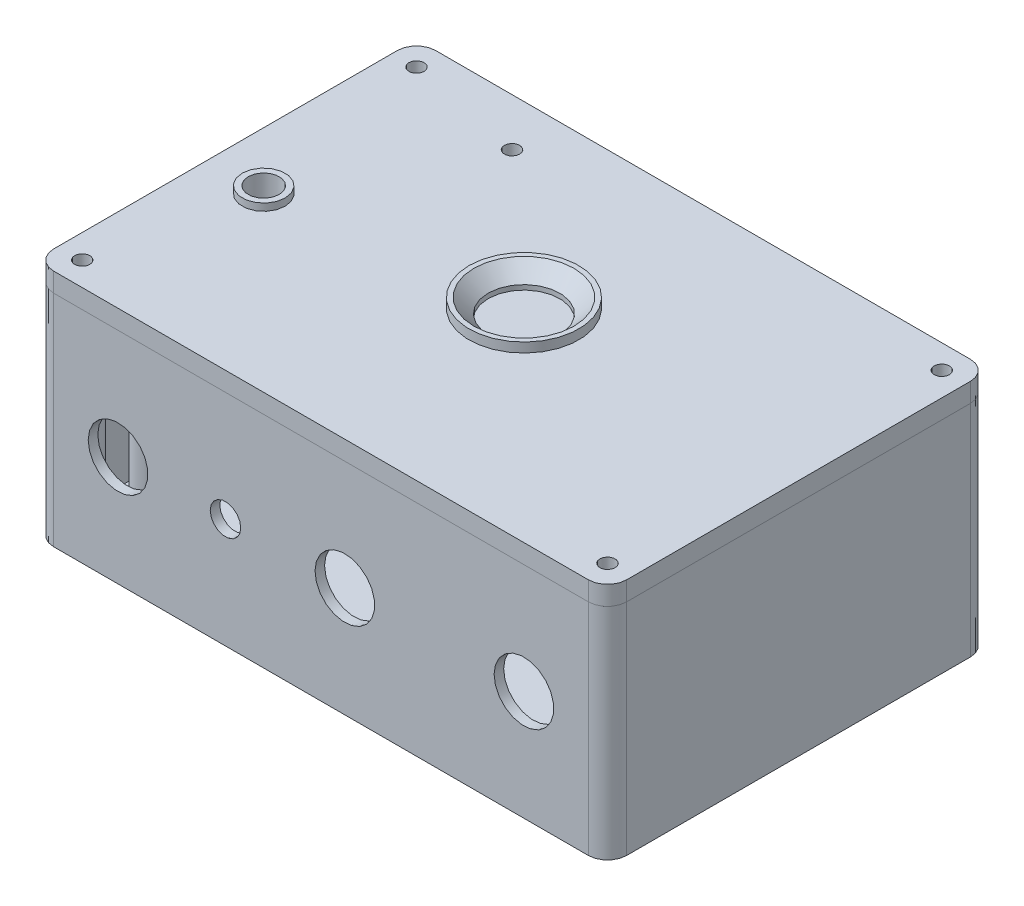
GridUp-Kutu (Autodesk Fusion 360 design; units mm, degrees)
part number: 2026-09-14-07-36-03-763
Autodesk Fusion 360 part; units mm, degrees
sketch "Çizim1" plane through (0, 0, 0) normal (0, 0, 1) x (1, 0, 0)
  line L0 (0, 0) -> (120, 0)
  line L1 (120, 0) -> (120, 80)
  line L2 (120, 80) -> (0, 80)
  line L3 (0, 80) -> (0, 0)
sketch "Çizim2" plane through (0, 0, 0) normal (0, 0, 1) x (1, 0, 0)
  circle A0 centre (5, 5) radius 3.5
  circle A1 centre (115, 5) radius 3.5
  circle A2 centre (5, 75) radius 3.5
  circle A3 centre (115, 75) radius 3.5
ref_plane "WorkPlane1" through (0, 0, 46) normal (0, 0, 1) x (1, 0, 0)
sketch "Çizim3" plane through (0, 0, 46) normal (0, 0, 1) x (1, 0, 0)
  line L0 (0, 0) -> (120, 0)
  line L1 (120, 0) -> (120, 80)
  line L2 (120, 80) -> (0, 80)
  line L3 (0, 80) -> (0, 0)
ref_plane "WorkPlane2" through (0, 0, 50) normal (0, 0, 1) x (1, 0, 0)
sketch "Çizim4" plane through (0, 0, 50) normal (0, 0, 1) x (1, 0, 0)
  circle A0 centre (60, 42.5) radius 11.5
sketch "Çizim5" plane through (0, 0, 50) normal (0, 0, 1) x (1, 0, 0)
  circle A0 centre (60, 42.5) radius 7.5
sketch "Çizim6" plane through (0, 0, 50) normal (0, 0, 1) x (1, 0, 0)
  circle A0 centre (12, 36) radius 4.5
sketch "Çizim7" plane through (0, 0, 50) normal (0, 0, 1) x (1, 0, 0)
  circle A0 centre (12, 36) radius 3.25
extrude "Ekstrüzyon7" cut sketch "Çizim7" along normal mid plane 16
sketch "Çizim8" plane through (0, 0, 50) normal (0, 0, 1) x (1, 0, 0)
  circle A0 centre (30, 70) radius 1.6
extrude "Ekstrüzyon8" cut sketch "Çizim8" along normal mid plane 16
sketch "Çizim9" plane through (0, 0, 50) normal (0, 0, 1) x (1, 0, 0)
  circle A0 centre (5, 5) radius 1.6
  circle A1 centre (115, 5) radius 1.6
  circle A2 centre (5, 75) radius 1.6
  circle A3 centre (115, 75) radius 1.6
extrude "Ekstrüzyon9" cut sketch "Çizim9" along normal mid plane 16
sketch "Çizim10" plane through (0, 0, 50) normal (0, 0, 1) x (1, 0, 0)
  circle A0 centre (5, 5) radius 1.25
  circle A1 centre (115, 5) radius 1.25
  circle A2 centre (5, 75) radius 1.25
  circle A3 centre (115, 75) radius 1.25
ref_plane "WorkPlane3" through (0, 0, 47.5) normal (0, 0, 1) x (1, 0, 0)
sketch "Çizim11" plane through (0, 0, 47.5) normal (0, 0, 1) x (1, 0, 0)
  circle A0 centre (60, 42.5) radius 7.5
sketch "Çizim12" plane through (0, 0, 0) normal (0, 1, 0) x (1, 0, 0)
  circle A0 centre (17.5, -23) radius 6.25
  circle A1 centre (47.5, -23) radius 5.5
  circle A2 centre (75, -23) radius 5.5
  circle A3 centre (102.5, -23) radius 3.2
sketch "Çizim13" plane through (0, 0, 0) normal (0, 0, 1) x (1, 0, 0)
  line L0 (12.75, 42.5) -> (22.25, 42.5)
  arc A0 (22.25, 42.5) -> (22.25, 48) centre (22.25, 45.25) ccw
  line L1 (22.25, 48) -> (12.75, 48)
  arc A1 (12.75, 48) -> (12.75, 42.5) centre (12.75, 45.25) ccw
  line L2 (97.75, 42.5) -> (107.25, 42.5)
  arc A2 (107.25, 42.5) -> (107.25, 48) centre (107.25, 45.25) ccw
  line L3 (107.25, 48) -> (97.75, 48)
  arc A3 (97.75, 48) -> (97.75, 42.5) centre (97.75, 45.25) ccw
sketch "Çizim14" plane through (0, 0, 0) normal (0, 0, 1) x (1, 0, 0)
  circle A0 centre (7.5, 7.5) radius 3.5
  circle A1 centre (112.5, 7.5) radius 3.5
  circle A2 centre (7.5, 72.5) radius 3.5
  circle A3 centre (112.5, 72.5) radius 3.5
sketch "Çizim15" plane through (0, 0, 0) normal (0, 0, 1) x (1, 0, 0)
  line L0 (42.5, 20) -> (77.5, 20)
  line L1 (77.5, 20) -> (77.5, 62)
  line L2 (77.5, 62) -> (42.5, 62)
  line L3 (42.5, 62) -> (42.5, 20)
ref_plane "WorkPlane4" through (0, 0, -5) normal (0, 0, 1) x (1, 0, 0)
sketch "Çizim16" plane through (0, 0, -5) normal (0, 0, 1) x (1, 0, 0)
  line L0 (42.5, 23.25) -> (77.5, 23.25)
  line L1 (77.5, 23.25) -> (77.5, 58.75)
  line L2 (77.5, 58.75) -> (42.5, 58.75)
  line L3 (42.5, 58.75) -> (42.5, 23.25)
sketch "Çizim17" plane through (0, 0, 0) normal (0, 0, 1) x (1, 0, 0)
  line L0 (0, 0) -> (120, 0)
  line L1 (120, 0) -> (120, 80)
  line L2 (120, 80) -> (0, 80)
  line L3 (0, 80) -> (0, 0)
sketch "Çizim18" plane through (0, 0, 0) normal (0, 0, 1) x (1, 0, 0)
  circle A0 centre (5, 5) radius 3.5
  circle A1 centre (115, 5) radius 3.5
  circle A2 centre (5, 75) radius 3.5
  circle A3 centre (115, 75) radius 3.5
sketch "Çizim19" plane through (0, 0, 0) normal (0, 0, 1) x (1, 0, 0)
  circle A0 centre (12, 12) radius 3
  circle A1 centre (108, 12) radius 3
  circle A2 centre (12, 68) radius 3
  circle A3 centre (108, 68) radius 3
ref_plane "WorkPlane5" through (0, 0, 39.4) normal (0, 0, 1) x (1, 0, 0)
sketch "Çizim20" plane through (0, 0, 39.4) normal (0, 0, 1) x (1, 0, 0)
  circle A0 centre (12, 12) radius 1.25
  circle A1 centre (108, 12) radius 1.25
  circle A2 centre (12, 68) radius 1.25
  circle A3 centre (108, 68) radius 1.25
ref_plane "WorkPlane6" through (0, 0, 46) normal (0, 0, 1) x (1, 0, 0)
sketch "Çizim21" plane through (0, 0, 46) normal (0, 0, 1) x (1, 0, 0)
  line L0 (0, 0) -> (120, 0)
  line L1 (120, 0) -> (120, 80)
  line L2 (120, 80) -> (0, 80)
  line L3 (0, 80) -> (0, 0)
extrude "Ekstrüzyon21" add sketch "Çizim21" along normal blind 4 separate body makes body 1
fillet "Radyus4" radius 4 4 edges at (0, 80, 48) (120, 80, 48) (120, 0, 48) (0, 0, 48) on bodies 1
ref_plane "WorkPlane7" through (0, 0, 50) normal (0, 0, 1) x (1, 0, 0)
sketch "Çizim22" plane through (0, 0, 50) normal (0, 0, 1) x (1, 0, 0)
  circle A0 centre (60, 42.5) radius 11.5
extrude "Ekstrüzyon22" add sketch "Çizim22" along normal blind 2 bodies 1
sketch "Çizim23" plane through (0, 0, 50) normal (0, 0, 1) x (1, 0, 0)
  circle A0 centre (60, 42.5) radius 7.5
extrude "Ekstrüzyon23" cut sketch "Çizim23" along normal mid plane 16 bodies 1
chamfer "Pah2" distance 3 angle 45 1 edges at (53.0075, 45.2121, 52) tangent chain off on bodies 1
sketch "Çizim24" plane through (0, 0, 50) normal (0, 0, 1) x (1, 0, 0)
  circle A0 centre (12, 36) radius 4.5
extrude "Ekstrüzyon24" add sketch "Çizim24" along normal blind 1.5 bodies 1
sketch "Çizim25" plane through (0, 0, 50) normal (0, 0, 1) x (1, 0, 0)
  circle A0 centre (12, 36) radius 3.25
extrude "Ekstrüzyon25" cut sketch "Çizim25" along normal mid plane 16 bodies 1
sketch "Çizim26" plane through (0, 0, 50) normal (0, 0, 1) x (1, 0, 0)
  circle A0 centre (30, 70) radius 1.6
extrude "Ekstrüzyon26" cut sketch "Çizim26" along normal mid plane 16 bodies 1
sketch "Çizim27" plane through (0, 0, 50) normal (0, 0, 1) x (1, 0, 0)
  circle A0 centre (5, 5) radius 1.6
  circle A1 centre (115, 5) radius 1.6
  circle A2 centre (5, 75) radius 1.6
  circle A3 centre (115, 75) radius 1.6
extrude "Ekstrüzyon27" cut sketch "Çizim27" along normal mid plane 16 bodies 1
sketch "Çizim28" plane through (0, 0, 50) normal (0, 0, 1) x (1, 0, 0)
  circle A0 centre (5, 5) radius 1.25
  circle A1 centre (115, 5) radius 1.25
  circle A2 centre (5, 75) radius 1.25
  circle A3 centre (115, 75) radius 1.25
ref_plane "WorkPlane8" through (0, 0, 47.5) normal (0, 0, 1) x (1, 0, 0)
sketch "Çizim29" plane through (0, 0, 47.5) normal (0, 0, 1) x (1, 0, 0)
  circle A0 centre (60, 42.5) radius 7.5
sketch "Çizim30" plane through (0, 0, 0) normal (0, 1, 0) x (1, 0, 0)
  circle A0 centre (17.5, -23) radius 6.25
  circle A1 centre (47.5, -23) radius 5.5
  circle A2 centre (75, -23) radius 5.5
  circle A3 centre (102.5, -23) radius 3.2
sketch "Çizim31" plane through (0, 0, 0) normal (0, 0, 1) x (1, 0, 0)
  line L0 (12.75, 42.5) -> (22.25, 42.5)
  arc A0 (22.25, 42.5) -> (22.25, 48) centre (22.25, 45.25) ccw
  line L1 (22.25, 48) -> (12.75, 48)
  arc A1 (12.75, 48) -> (12.75, 42.5) centre (12.75, 45.25) ccw
  line L2 (97.75, 42.5) -> (107.25, 42.5)
  arc A2 (107.25, 42.5) -> (107.25, 48) centre (107.25, 45.25) ccw
  line L3 (107.25, 48) -> (97.75, 48)
  arc A3 (97.75, 48) -> (97.75, 42.5) centre (97.75, 45.25) ccw
sketch "Çizim32" plane through (0, 0, 0) normal (0, 0, 1) x (1, 0, 0)
  circle A0 centre (7.5, 7.5) radius 3.5
  circle A1 centre (112.5, 7.5) radius 3.5
  circle A2 centre (7.5, 72.5) radius 3.5
  circle A3 centre (112.5, 72.5) radius 3.5
sketch "Çizim33" plane through (0, 0, 0) normal (0, 0, 1) x (1, 0, 0)
  line L0 (42.5, 20) -> (77.5, 20)
  line L1 (77.5, 20) -> (77.5, 62)
  line L2 (77.5, 62) -> (42.5, 62)
  line L3 (42.5, 62) -> (42.5, 20)
ref_plane "WorkPlane9" through (0, 0, -5) normal (0, 0, 1) x (1, 0, 0)
sketch "Çizim34" plane through (0, 0, -5) normal (0, 0, 1) x (1, 0, 0)
  line L0 (42.5, 23.25) -> (77.5, 23.25)
  line L1 (77.5, 23.25) -> (77.5, 58.75)
  line L2 (77.5, 58.75) -> (42.5, 58.75)
  line L3 (42.5, 58.75) -> (42.5, 23.25)
sketch "Çizim35" plane through (0, 0, 0) normal (0, 0, 1) x (1, 0, 0)
  line L0 (0, 0) -> (120, 0)
  line L1 (120, 0) -> (120, 80)
  line L2 (120, 80) -> (0, 80)
  line L3 (0, 80) -> (0, 0)
extrude "Ekstrüzyon35" add sketch "Çizim35" along normal blind 46 separate body makes body 2
fillet "Radyus5" radius 4 4 edges at (0, 80, 23) (120, 80, 23) (120, 0, 23) (0, 0, 23) on bodies 2
shell "Kabuk3" thickness 2 removed faces 1 at (78.6667, 26.6667, 46) on bodies 2
sketch "Çizim36" plane through (0, 0, 0) normal (0, 0, 1) x (1, 0, 0)
  circle A0 centre (5, 5) radius 3.5
  circle A1 centre (115, 5) radius 3.5
  circle A2 centre (5, 75) radius 3.5
  circle A3 centre (115, 75) radius 3.5
extrude "Ekstrüzyon36" add sketch "Çizim36" along normal blind 46 bodies 2
sketch "Çizim37" plane through (0, 0, 0) normal (0, 0, 1) x (1, 0, 0)
  circle A0 centre (12, 12) radius 3
  circle A1 centre (108, 12) radius 3
  circle A2 centre (12, 68) radius 3
  circle A3 centre (108, 68) radius 3
extrude "Ekstrüzyon37" add sketch "Çizim37" along normal blind 39.4 bodies 2
ref_plane "WorkPlane10" through (0, 0, 39.4) normal (0, 0, 1) x (1, 0, 0)
sketch "Çizim38" plane through (0, 0, 39.4) normal (0, 0, 1) x (1, 0, 0)
  circle A0 centre (12, 12) radius 1.25
  circle A1 centre (108, 12) radius 1.25
  circle A2 centre (12, 68) radius 1.25
  circle A3 centre (108, 68) radius 1.25
extrude "Ekstrüzyon38" cut sketch "Çizim38" against normal blind 8 bodies 2
ref_plane "WorkPlane11" through (0, 0, 46) normal (0, 0, 1) x (1, 0, 0)
sketch "Çizim39" plane through (0, 0, 46) normal (0, 0, 1) x (1, 0, 0)
  line L0 (0, 0) -> (120, 0)
  line L1 (120, 0) -> (120, 80)
  line L2 (120, 80) -> (0, 80)
  line L3 (0, 80) -> (0, 0)
extrude "Ekstrüzyon39" add sketch "Çizim39" along normal blind 4 separate body makes body 3
fillet "Radyus6" radius 4 4 edges at (0, 80, 48) (120, 80, 48) (120, 0, 48) (0, 0, 48) on bodies 3
ref_plane "WorkPlane12" through (0, 0, 50) normal (0, 0, 1) x (1, 0, 0)
sketch "Çizim40" plane through (0, 0, 50) normal (0, 0, 1) x (1, 0, 0)
  circle A0 centre (60, 42.5) radius 11.5
extrude "Ekstrüzyon40" add sketch "Çizim40" along normal blind 2 bodies 3
sketch "Çizim41" plane through (0, 0, 50) normal (0, 0, 1) x (1, 0, 0)
  circle A0 centre (60, 42.5) radius 7.5
extrude "Ekstrüzyon41" cut sketch "Çizim41" along normal mid plane 16 bodies 3
chamfer "Pah3" distance 3 angle 45 1 edges at (53.0075, 45.2121, 52) tangent chain off on bodies 3
sketch "Çizim42" plane through (0, 0, 50) normal (0, 0, 1) x (1, 0, 0)
  circle A0 centre (12, 36) radius 4.5
extrude "Ekstrüzyon42" add sketch "Çizim42" along normal blind 1.5 bodies 3
sketch "Çizim43" plane through (0, 0, 50) normal (0, 0, 1) x (1, 0, 0)
  circle A0 centre (12, 36) radius 3.25
extrude "Ekstrüzyon43" cut sketch "Çizim43" along normal mid plane 16 bodies 3
sketch "Çizim44" plane through (0, 0, 50) normal (0, 0, 1) x (1, 0, 0)
  circle A0 centre (30, 70) radius 1.6
extrude "Ekstrüzyon44" cut sketch "Çizim44" along normal mid plane 16 bodies 3
sketch "Çizim45" plane through (0, 0, 50) normal (0, 0, 1) x (1, 0, 0)
  circle A0 centre (5, 5) radius 1.6
  circle A1 centre (115, 5) radius 1.6
  circle A2 centre (5, 75) radius 1.6
  circle A3 centre (115, 75) radius 1.6
extrude "Ekstrüzyon45" cut sketch "Çizim45" along normal mid plane 16 bodies 3
sketch "Çizim46" plane through (0, 0, 50) normal (0, 0, 1) x (1, 0, 0)
  circle A0 centre (5, 5) radius 1.25
  circle A1 centre (115, 5) radius 1.25
  circle A2 centre (5, 75) radius 1.25
  circle A3 centre (115, 75) radius 1.25
extrude "Ekstrüzyon46" cut sketch "Çizim46" against normal blind 16 bodies 2
ref_plane "WorkPlane13" through (0, 0, 47.5) normal (0, 0, 1) x (1, 0, 0)
sketch "Çizim47" plane through (0, 0, 47.5) normal (0, 0, 1) x (1, 0, 0)
  circle A0 centre (60, 42.5) radius 7.5
extrude "Ekstrüzyon47" add sketch "Çizim47" along normal mid plane 1 separate body makes body 4
sketch "Çizim48" plane through (0, 0, 0) normal (0, 1, 0) x (1, 0, 0)
  circle A0 centre (17.5, -23) radius 6.25
  circle A1 centre (40, -23) radius 3.2
  circle A2 centre (65, -23) radius 6.25
  circle A3 centre (102.5, -23) radius 6.25
extrude "Ekstrüzyon48" cut sketch "Çizim48" along normal mid plane 6 bodies 2
sketch "Çizim49" plane through (0, 0, 0) normal (0, 0, 1) x (1, 0, 0)
  line L0 (12.75, 42.5) -> (22.25, 42.5)
  arc A0 (22.25, 42.5) -> (22.25, 48) centre (22.25, 45.25) ccw
  line L1 (22.25, 48) -> (12.75, 48)
  arc A1 (12.75, 48) -> (12.75, 42.5) centre (12.75, 45.25) ccw
  line L2 (97.75, 42.5) -> (107.25, 42.5)
  arc A2 (107.25, 42.5) -> (107.25, 48) centre (107.25, 45.25) ccw
  line L3 (107.25, 48) -> (97.75, 48)
  arc A3 (97.75, 48) -> (97.75, 42.5) centre (97.75, 45.25) ccw
extrude "Ekstrüzyon49" cut sketch "Çizim49" along normal mid plane 6 bodies 2
sketch "Çizim50" plane through (0, 0, 0) normal (0, 0, 1) x (1, 0, 0)
  circle A0 centre (7.5, 7.5) radius 3.5
  circle A1 centre (112.5, 7.5) radius 3.5
  circle A2 centre (7.5, 72.5) radius 3.5
  circle A3 centre (112.5, 72.5) radius 3.5
extrude "Ekstrüzyon50" cut sketch "Çizim50" along normal mid plane 2 bodies 2
sketch "Çizim51" plane through (0, 0, 0) normal (0, 0, 1) x (1, 0, 0)
  line L0 (42.5, 20) -> (77.5, 20)
  line L1 (77.5, 20) -> (77.5, 62)
  line L2 (77.5, 62) -> (42.5, 62)
  line L3 (42.5, 62) -> (42.5, 20)
extrude "Ekstrüzyon51" add sketch "Çizim51" against normal blind 5 separate body makes body 5
ref_plane "WorkPlane14" through (0, 0, -5) normal (0, 0, 1) x (1, 0, 0)
sketch "Çizim52" plane through (0, 0, -5) normal (0, 0, 1) x (1, 0, 0)
  line L0 (42.5, 23.25) -> (77.5, 23.25)
  line L1 (77.5, 23.25) -> (77.5, 58.75)
  line L2 (77.5, 58.75) -> (42.5, 58.75)
  line L3 (42.5, 58.75) -> (42.5, 23.25)
extrude "Ekstrüzyon52" cut sketch "Çizim52" along normal mid plane 6 bodies 5
hidden bodies 3
equation "d110 = -( 8 mm )"
equation "d133 = -( 16 mm )"
equation "d145 = -( 5 mm )"
named bodies: "Kapak", "Gövde", "Kapak (1)", "IR pencere", "DIN klips"
